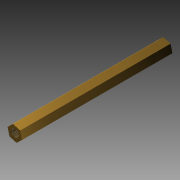
# Autodesk Inventor part: Spacer60
Saved by Autodesk Inventor 2015 (Build 190159000, 159)
## iProperties
Created: 2015-10-11
Part Number: Spacer60
Material: Generic
Document SubType Name: Modeling
Designer: styku
Density: 1 g/cm^3
Appearance: Brass - Polished
Mass: 0.978846 g
Surface Area: 16.7811 cm^2
Volume: 0.978846 cm^3
Author: styku
Autodesk Inventor part; units mm, degrees
ref_plane "YZ Plane" through (0, 0, 0) normal (1, 0, 0) x (0, 1, 0)
ref_plane "XZ Plane" through (0, 0, 0) normal (0, 1, 0) x (-1, 0, 0)
ref_plane "XY Plane" through (0, 0, 0) normal (0, 0, 1) x (1, 0, 0)
sketch "Sketch1" plane through (0, 0, 0) normal (0, 1, 0) x (-1, 0, 0)
  circle A0 centre (0, 0) radius 1.5
  line L0 (-0.7211, -2.912) -> (-2.8825, -0.8315)
  line L1 (-2.8825, -0.8315) -> (-2.1614, 2.0805)
  line L2 (-2.1614, 2.0805) -> (0.7211, 2.912)
  line L3 (0.7211, 2.912) -> (2.8825, 0.8315)
  line L4 (2.8825, 0.8315) -> (2.1614, -2.0805)
  line L5 (2.1614, -2.0805) -> (-0.7211, -2.912)
  dimension "d0" = 3
  dimension "d1" = 6
  constraints: 12 end point, 2 coincident, 1 centre point, 13 other
  measures "d0" diameter of A0
  measures "d1" distance of L2.end L0.start
extrude "Extrusion1" add sketch "Sketch1" along normal blind 60
thread "Thread1" size "M3x0.5" class "6H" standard "ANSI Metric M Profile" length 10
thread "Thread2" size "M3x0.5" class "6H" standard "ANSI Metric M Profile" length 10
body "Solid1"
